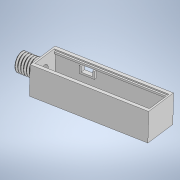
# Autodesk Inventor part: battery and buck converter enclosure
Saved by Autodesk Inventor 2022 (Build 260153000, 153)
## iProperties
Created: 2021-10-07
Part Number: battery and buck converter enclosure
Material: Generic
Document SubType Name: Modeling
Designer: tecware
Density: 1 g/cm^3
Appearance: Default
Author: tecware
## iProperties of the stored document battery and buck converter enclosure_3DPrint.ipt
Created: 2021-10-07
Part Number: battery and buck converter enclosure_3DPrint
Material: Generic
Document SubType Name: Modeling
Designer: tecware
Density: 1 g/cm^3
Appearance: Default
Author: tecware
Autodesk Inventor part; units mm, degrees
ref_plane "YZ Plane" through (0, 0, 0) normal (1, 0, 0) x (0, 1, 0)
ref_plane "XZ Plane" through (0, 0, 0) normal (0, 1, 0) x (-1, 0, 0)
ref_plane "XY Plane" through (0, 0, 0) normal (0, 0, 1) x (1, 0, 0)
sketch "Sketch1" plane through (0, 0, 0) normal (0, 1, 0) x (-1, 0, 0)
  line L0 (90, -17.5) -> (-30, -17.5)
  line L1 (-30, -17.5) -> (-30, 15.5)
  line L2 (-30, 15.5) -> (90, 15.5)
  line L3 (90, 15.5) -> (90, -17.5)
  dimension "d0" = 120
  dimension "d1" = 33
  constraints: 8 end point, 2 parallel, 1 horizontal, 1 perpendicular
  measures "d0" distance of L1.end L2.end
  measures "d1" distance of L0.end L1.end
extrude "Main Body" add sketch "Sketch1" along normal blind 30
shell "Main Shell" thickness 2 outward yes removed faces 1 at (-50, 30, -6.5)
sketch "Sketch19" plane through (-90, 0, -17.5) normal (1, 0, 0) x (0, 0, -1)
  line L0 (-33, 30) -> (-33, 27)
  line L1 (-33, 30) -> (-31, 30)
  line L2 (2, 30) -> (-35, 30) projected
  line L3 (-33, 27) -> (-31, 30)
  line L4 (-16.5, 30) -> (-16.5, 25)
  line L5 (-33, 27) -> (-31, 27)
  line L6 (-31, 27) -> (-31, 25)
  line L7 (-31, 25) -> (-33, 25)
  line L8 (-33, 25) -> (-33, 27)
  line L9 (0, 0) -> (-33, 0) projected
  line L10 (0, 0) -> (0, 30) projected
  line L11 (-33, 30) -> (0, 30) projected
  line L12 (-33, 0) -> (-33, 30) projected
  line L13 (0, 30) -> (0, 27)
  line L14 (0, 30) -> (-2, 30)
  line L15 (0, 27) -> (-2, 30)
  line L16 (0, 27) -> (-2, 27)
  line L17 (-2, 27) -> (-2, 25)
  line L18 (-2, 25) -> (0, 25)
  line L19 (0, 25) -> (0, 27)
  point P0 (-17.5, 0)
  point P1 (-33, 28.5)
  point P2 (0, 28.5)
  dimension "d107" = 2
  dimension "d108" = 3
  dimension "d109" = 2
  dimension "d110" = 2
  constraints: 30 end point, 8 symmetric about line, 2 midpoint, 2 parallel, 2 point on line, 2 vertical, 1 horizontal, 1 perpendicular
  measures "d107" distance of L0.start L1.end
  measures "d108" distance of L0.start L0.end
  measures "d109" distance of L7.end L0.end
  measures "d110" distance of L6.end L7.end
extrude "Rail" add sketch "Sketch19" along normal up to surface (122 mm away) contours L1 L3 L0 | L5 L6 L7 L8 | L2 L10 L15 | L10 L18 L17 L16
sketch "Sketch3" plane through (-90, 0, -17.5) normal (0, 0, 1) x (1, 0, 0)
  line L0 (29, 24) -> (41.1, 24)
  line L1 (41.1, 24) -> (41.1, 18)
  line L2 (41.1, 18) -> (29, 18)
  line L3 (29, 18) -> (29, 24)
  line L4 (0, 30) -> (120, 30) projected
  point P0 (90, 0)
  dimension "d9" = 12.1
  dimension "d10" = 6
  dimension "d75" = 6
  constraints: 8 end point, 2 parallel, 1 horizontal, 1 perpendicular
  measures "d9" distance of L1.end L2.end
  measures "d10" distance of L0.end L1.end
  measures "d75" distance between parallel lines of L4 L0
extrude "Switch Cutout" cut sketch "Sketch3" along normal mid plane 16
sketch "Sketch8" plane through (-90, 0, -17.5) normal (0, 0, 1) x (1, 0, 0)
  line L0 (29, 18) -> (41.1, 18) projected
  line L1 (29, 30) -> (41.1, 30)
  line L2 (41.1, 30) -> (41.1, 18)
  line L3 (41.1, 18) -> (29, 18)
  line L4 (29, 18) -> (29, 30)
  line L5 (27, 30) -> (43.1, 30)
  line L6 (43.1, 30) -> (43.1, 16)
  line L7 (43.1, 16) -> (27, 16)
  line L8 (27, 16) -> (27, 30)
  line L9 (27, 24) -> (43.1, 24)
  point P0 (90, 0)
  point P1 (41.1, 24)
  point P2 (29, 24)
  dimension "d40" = 2
  dimension "d41" = 2
  dimension "d42" = 2
  dimension "d77" = 6
  constraints: 18 end point, 4 parallel, 3 perpendicular, 2 horizontal, 2 point on line
  measures "d40" distance between parallel lines of L4 L8
  measures "d41" distance between parallel lines of L6 L2
  measures "d42" distance between parallel lines of L0 L7
  measures "d77" distance between parallel lines of L9 L0
extrude "Switch Holder" add sketch "Sketch8" along normal blind 3 contours L0 L2 L9 L6 L7 L8 L4
sketch "Sketch9" plane through (-92, -2, -19.5) normal (-1, 0, 0) x (0, 0, 1)
  circle A0 centre (18.5, 17) radius 6
  circle A1 centre (18.5, 17) radius 8
  line L0 (35, 2) -> (35, 32) projected
  line L1 (2, 2) -> (35, 2) projected
  point P0 (19.5, 2)
  dimension "d45" = 12
  dimension "d46" = 16
  dimension "d78" = 16.5
  dimension "d79" = 15
  constraints: 2 centre point, 1 coincident
  measures "d45" diameter of A0
  measures "d46" diameter of A1
  measures "d78" distance from line of L0 A0.centre
  measures "d79" distance from line of L1 A0.centre
extrude "Raised" add sketch "Sketch9" along normal blind 3
sketch "thread" plane through (-95, 2, -18.5) normal (-1, 0, 0) x (0, 0, 1)
  circle A0 centre (17.5, 13) radius 6
  circle A1 centre (17.5, 13) radius 10
  point P0 (18.5, -2)
  dimension "d13" = 12
  dimension "d14" = 20
  constraints: 2 centre point, 2 coincident
  measures "d13" diameter of A0
  measures "d14" diameter of A1
extrude "Extrusion10" add sketch "thread" along normal blind 20 contours A0 | A1
sketch "Sketch13" plane through (-90, 15, -2) normal (-1, 0, 0) x (0, 0, 1)
  circle A0 centre (1, 0) radius 6
  line L0 (-15.5, -15) -> (-15.5, 10) projected
  line L1 (-15.5, -15) -> (17.5, -15) projected
  point P0 (2, -15)
  dimension "d72" = 12
  dimension "d112" = 16.5
  dimension "d113" = 15
  constraints: 1 centre point
  measures "d72" diameter of A0
  measures "d112" distance from line of L0 A0.centre
  measures "d113" distance from line of L1 A0.centre
extrude "Through Hole For Wire" cut sketch "Sketch13" along normal through all
thread "Thread4" size "M22x3" class "6g" standard "ANSI Metric M Profile" full length
sketch "Sketch21" plane through (-115, 15, -1) normal (0, 1, 0) x (0, 0, 1)
  line L0 (10, 0) -> (10, 20)
  line L1 (10, 20) -> (7.7756, 20)
  line L2 (7.7756, 20) -> (7.7756, 0)
  line L3 (7.7756, 0) -> (10, 0)
  line L4 (0, -33.3256) -> (0, 177.0543) projected
  constraints: 8 end point
revolve "Revolution7" cut sketch "Sketch21" angle 360 about axis through (-115, 15, -1) along (1, 0, 0)
sketch "Sketch22" plane through (-115, 15, -1) normal (0, 1, 0) x (0, 0, 1)
  line L0 (10, 0) -> (10, 20)
  line L1 (10, 20) -> (7.7756, 20)
  line L2 (7.7756, 20) -> (7.7756, 0)
  line L3 (7.7756, 0) -> (10, 0)
  line L4 (0, -33.3256) -> (0, 177.0543) projected
  constraints: 8 end point
revolve "Revolution8" add sketch "Sketch22" angle 360 about axis through (-115, 15, -1) along (1, 0, 0) separate body
sketch "Sketch20" plane through (-115, 15, -1) normal (0, -1, 0) x (1, 0, 0)
  line L0 (-1.7501, -7.9275) -> (-1.5001, -7.9275) construction
  line L1 (0.2499, -9.8485) -> (-0.0001, -10.3287) construction
  line L2 (-3.0001, -10.3287) -> (-3.2501, -9.8485) construction
  line L3 (-1.2501, -7.9275) -> (-1.5001, -7.4472) construction
  line L4 (-1.5001, -7.4472) -> (-1.7501, -7.9275) construction
  line L5 (-3.0001, -10.3287) -> (-2.7501, -9.8485) construction
  line L6 (-1.2501, -7.9275) -> (-0.2501, -9.8485)
  line L7 (-3.2501, -9.8485) -> (-2.7501, -9.8485) construction
  arc A0 (-3.2501, -9.8485) -> (-3.0001, -10.0002) centre (-3.0001, -9.7183) ccw construction
  line L8 (0.2499, -9.8485) -> (-0.2501, -9.8485) construction
  line L9 (-3.0001, -10.3287) -> (-3.0001, -9.8485) construction
  line L10 (-0.0001, -10.3287) -> (-0.0001, -9.8485) construction
  line L11 (-1.5001, -7.4472) -> (-1.5001, -7.7758) construction
  line L12 (-3.0001, -10.0002) -> (-0.0001, -10.0002)
  arc A1 (-3.0001, -10.0002) -> (-2.7501, -9.8485) centre (-3.0001, -9.7183) ccw
  line L13 (-0.2501, -9.8485) -> (-0.0001, -10.3287) construction
  line L14 (-2.7501, -9.8485) -> (-1.7501, -7.9275)
  line L15 (-0.0001, -0.0002) -> (-0.0001, 0.0177)
  line L16 (-0.0001, 0.0177) -> (-0.0001, -0.0002)
  line L17 (-0.0001, -0.0002) -> (0.0334, -0.0002)
  arc A2 (-0.2501, -9.8485) -> (-0.0001, -10.0002) centre (-0.0001, -9.7183) ccw
  arc A3 (-0.0001, -10.0002) -> (0.2499, -9.8485) centre (-0.0001, -9.7183) ccw construction
  arc A4 (-1.5001, -7.7758) -> (-1.7501, -7.9275) centre (-1.5001, -8.0576) ccw
  arc A5 (-1.2501, -7.9275) -> (-1.5001, -7.7758) centre (-1.5001, -8.0576) ccw
  line L18 (-1.5001, -7.7758) -> (-1.5001, -7.9275) construction
  line L19 (-1.5001, -7.9275) -> (-1.2501, -7.9275) construction
  dimension "d116" = 55
  dimension "d117" = 0.4803
  dimension "d118" = 0.4803
  dimension "Sketch20_ThreadOffset" = 0
  dimension "Sketch20_MajorRadius" = 10
  dimension "d121" = 3
  dimension "Sketch20_MinorRadius" = 7.7756
  constraints: 40 end point, 12 point on circle, 10 parallel, 8 tangent, 6 centre point, 6 collinear, 2 midpoint, 2 point on line, 1 horizontal, 1 perpendicular, 3 other
  measures "d116" angle of L6 L14
  measures "d117" distance of L3.end L0.end
  measures "d118" distance of L1.end L10.end
  measures "Sketch20_ThreadOffset" distance between parallel lines of L15 L10
  measures "Sketch20_MajorRadius" distance from line of L12 L15.start
  measures "d121" distance from line of L1.end L9
  measures "Sketch20_MinorRadius" distance edge to line of A5 L17
coil "Coil4" sketch "Sketch20" operation cut axis through (-115, 15, -1) along (1, 0, 0) pitch 3.003 turns 8.658009 hand right bodies 2
combine bodies "Combine1" operation type add bodies to combine 1 2
equation "\"d109\" = d107"
equation "\"d110\" = d107"
equation "\"d41\" = d40"
equation "\"d42\" = d40"
equation "\"d78\" = 0.5 * d1"
equation "\"d79\" = 0.5 * d2"
equation "\"d112\" = 0.5 * d1"
equation "\"d113\" = 0.5 * d2"
equation "\"d116\" = d123"
equation "\"d117\" = 0.160083 * Sketch20_Pitch"
equation "\"d118\" = 0.160083 * Sketch20_Pitch"
equation "\"d121\" = Sketch20_Pitch"
equation "\"d28\" = 55deg"
equation "\"Sketch5_Pitch\" = 3"
equation "\"d60\" = 55deg"
equation "\"Sketch10_Pitch\" = 3"
equation "\"d91\" = 55deg"
equation "\"Sketch14_Pitch\" = 3"
equation "\"d123\" = 55deg"
equation "\"Sketch20_Pitch\" = 3"
equation "\"d2\" = 30"
body "Solid5"
